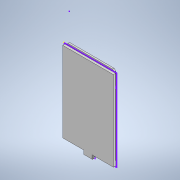
# Autodesk Inventor part: Main_Housing_Cap
Saved by Autodesk Inventor 2021 (Build 250183000, 183)
## iProperties
Created: 2020-12-01
Part Number: Main_Housing_Cap
Material: Generic
Document SubType Name: Modeling
Designer: Blake
Density: 1 g/cm^3
Appearance: Default
Author: Blake
Autodesk Inventor part; units mm, degrees
ref_plane "YZ Plane" through (0, 0, 0) normal (1, 0, 0) x (0, 1, 0)
ref_plane "XZ Plane" through (0, 0, 0) normal (0, 1, 0) x (-1, 0, 0)
ref_plane "XY Plane" through (0, 0, 0) normal (0, 0, 1) x (1, 0, 0)
sketch "Sketch1" plane through (0, 0, 0) normal (0, 0, 1) x (1, 0, 0)
  line L0 (24.765, -64.933) -> (24.765, -65.405)
  line L1 (41.91, -65.405) -> (24.765, -65.405)
  line L2 (41.91, 0) -> (41.91, -65.405)
  line L3 (0, 0) -> (41.91, 0)
  line L4 (0, -65.405) -> (0, 0)
  line L5 (17.145, -65.405) -> (0, -65.405)
  line L6 (17.145, -65.405) -> (17.145, -64.933)
  line L7 (17.145, -64.933) -> (0.472, -64.933)
  line L8 (0.472, -64.933) -> (0.472, -0.472)
  line L9 (0.472, -0.472) -> (41.438, -0.472)
  line L10 (41.438, -0.472) -> (41.438, -64.933)
  line L11 (41.438, -64.933) -> (24.765, -64.933)
  line L12 (17.145, -64.933) -> (17.145, -63.6597)
  line L13 (17.145, -63.6597) -> (3.0153, -63.6597)
  arc A0 (1.7453, -62.3897) -> (3.0153, -63.6597) centre (3.0153, -62.3897) ccw
  line L14 (1.7453, -62.3897) -> (1.7453, -10.7786)
  arc A1 (1.7453, -10.7786) -> (0.472, -9.5086) centre (0.4753, -10.7786) ccw
  line L15 (0.472, -64.933) -> (0.472, -9.5086)
  line L16 (17.145, -64.933) -> (0.472, -64.933)
  line L17 (24.765, -63.6597) -> (24.765, -64.933)
  line L18 (41.438, -64.933) -> (24.765, -64.933)
  line L19 (41.438, -9.5086) -> (41.438, -64.933)
  arc A2 (41.438, -9.5086) -> (40.1647, -10.7786) centre (41.4347, -10.7786) ccw
  line L20 (40.1647, -10.7786) -> (40.1647, -62.3897)
  arc A3 (38.8947, -63.6597) -> (40.1647, -62.3897) centre (38.8947, -62.3897) ccw
  line L21 (38.8947, -63.6597) -> (24.765, -63.6597)
  line L22 (24.765, -67.945) -> (17.145, -67.945)
  line L23 (24.765, -63.6597) -> (24.765, -67.945)
  line L24 (17.145, -63.6597) -> (24.765, -63.6597)
  line L25 (17.145, -67.945) -> (17.145, -63.6597)
  point P0 (4.318, 23.368)
  constraints: 52 end point, 8 point on circle, 4 centre point
extrude "Extrusion1" add sketch "Sketch1" along normal blind 1.7526 contours L17 L21 A3 L20 A2 L10 L11 | L0 L23 L22 L25 L6 L12 L24 L17 | L24 L13 A0 L14 A1 L8 L9 L10 A2 L20 A3 L21 | L12 L7 L8 A1 L14 A0 L13
sketch "Sketch2" plane through (0, 0, 0) normal (0, 0, -1) x (-1, 0, 0)
  line L0 (-41.438, -0.472) -> (-0.472, -0.472) projected
  line L1 (-41.438, -64.933) -> (-41.438, -0.472) projected
  line L2 (-24.765, -64.933) -> (-41.438, -64.933) projected
  line L3 (-24.765, -67.945) -> (-24.765, -64.933) projected
  line L4 (-17.145, -67.945) -> (-24.765, -67.945) projected
  line L5 (-17.145, -64.933) -> (-17.145, -67.945) projected
  line L6 (-0.472, -64.933) -> (-17.145, -64.933) projected
  line L7 (-0.472, -0.472) -> (-0.472, -64.933) projected
  line L8 (-39.914, -61.885) -> (-39.914, -0.472)
  line L9 (-1.996, -0.472) -> (-1.996, -61.885)
  line L10 (-3.52, -63.409) -> (-38.39, -63.409)
  arc A0 (-39.914, -61.885) -> (-38.39, -63.409) centre (-38.39, -61.885) ccw
  arc A1 (-3.52, -63.409) -> (-1.996, -61.885) centre (-3.52, -61.885) ccw
  line L11 (-41.438, -0.472) -> (-0.472, -0.472) projected
  line L12 (-4.536, 2.068) -> (-37.374, 2.068)
  line L13 (-1.996, -0.472) -> (-1.996, -0.472)
  line L14 (-37.374, 2.068) -> (-39.914, -0.472)
  line L15 (-4.536, 2.068) -> (-1.996, -0.472)
  point P0 (0, 0)
  point P1 (-39.914, 2.068)
  point P2 (-1.996, 2.068)
  dimension "d2" = 1.524
  dimension "d3" = 1.524
  dimension "d4" = 1.524
  dimension "d5" = 1.524
  dimension "d7" = 2.54
  dimension "d8" = 2.54
  dimension "d9" = 2.54
  dimension "d10" = 2.54
  constraints: 14 end point, 4 point on circle, 4 point on line, 4 tangent, 3 parallel, 2 centre point, 1 equal radius, 1 horizontal, 1 vertical, 1 other
  measures "d2" distance between parallel lines of L1 L8
  measures "d3" distance between parallel lines of L7 L9
  measures "d4" distance between parallel lines of L2 L10
  measures "d5" radius of A0
  measures "d7" distance of L12.end point (-39.914, 2.068)
  measures "d8" distance of L8.end point (-39.914, 2.068)
  measures "d9" distance of L12.start point (-1.996, 2.068)
  measures "d10" distance of L13.end point (-1.996, 2.068)
extrude "Extrusion2" add sketch "Sketch2" along normal blind 1.27 contours L14 L12 L15 L0 | L0 L9 A1 L10 A0 L8
chamfer "Chamfer1" distance 1.27 angle 45 1 edges at (20.955, -67.945, 0)
sketch "Sketch3" plane through (0, 0, 1.7526) normal (0, 0, 1) x (1, 0, 0)
  line L0 (41.438, -0.472) -> (0.472, -0.472) projected
  line L1 (0.472, -0.472) -> (0.472, -64.933) projected
  line L2 (0.472, -64.933) -> (17.145, -64.933) projected
  line L3 (17.145, -64.933) -> (17.145, -67.945) projected
  line L4 (17.145, -67.945) -> (24.765, -67.945) projected
  line L5 (24.765, -67.945) -> (24.765, -64.933) projected
  line L6 (24.765, -64.933) -> (41.438, -64.933) projected
  line L7 (41.438, -64.933) -> (41.438, -0.472) projected
  line L8 (41.063, -0.847) -> (0.847, -0.847)
  line L9 (0.847, -0.847) -> (0.847, -64.558)
  line L10 (0.847, -64.558) -> (17.52, -64.558)
  line L11 (17.52, -64.558) -> (17.52, -67.57)
  line L12 (17.52, -67.57) -> (24.39, -67.57)
  line L13 (24.39, -67.57) -> (24.39, -64.558)
  line L14 (24.39, -64.558) -> (41.063, -64.558)
  line L15 (41.063, -64.558) -> (41.063, -0.847)
  point P0 (0, 0)
  constraints: 16 end point, 7 other
extrude "Extrusion3" cut sketch "Sketch3" against normal up to surface (1.7526 mm away)
sketch "Sketch4" plane through (0, 0, 0) normal (0, 0, 1) x (1, 0, 0)
  line L0 (37.374, 2.068) -> (39.914, -0.472) projected
  line L1 (4.536, 2.068) -> (37.374, 2.068) projected
  line L2 (1.996, -0.472) -> (4.536, 2.068) projected
  line L3 (1.996, -0.472) -> (1.996, -0.847) projected
  line L4 (1.996, -0.847) -> (39.914, -0.847) projected
  line L5 (39.914, -0.847) -> (39.914, -0.472) projected
  line L6 (1.996, -0.472) -> (4.536, 2.068) projected
  line L7 (3.266, 0.798) -> (38.644, 0.798)
  line L8 (38.644, 0.798) -> (38.644, 2.068)
  line L9 (38.644, 2.068) -> (3.266, 2.068)
  line L10 (3.266, 2.068) -> (3.266, 0.798)
  point P0 (0, 0)
  constraints: 8 end point, 2 parallel, 1 horizontal, 1 midpoint, 1 perpendicular
extrude "Extrusion4" cut sketch "Sketch4" against normal blind 1.27 contours L9 L8 L0 | L0 L7 L2 L1 | L2 L10 L9
equation "\"d8\" = d7"
equation "\"d9\" = d7"
equation "\"d10\" = d9"
body "Solid1"
